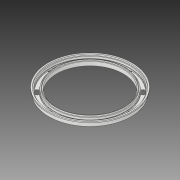
# Autodesk Inventor part: led_holster
Saved by Autodesk Inventor 2019.3 (Build 233278000, 278)
## iProperties
Created: 2019-03-01
Part Number: led_holster
Material: ABS Plastic
Document SubType Name: Modeling
Designer: WW
Density: 1.06 g/cm^3
Appearance: Smooth - White
Author: WW
Autodesk Inventor part; units mm, degrees
ref_plane "YZ Plane" through (0, 0, 0) normal (1, 0, 0) x (0, 1, 0)
ref_plane "XZ Plane" through (0, 0, 0) normal (0, 1, 0) x (-1, 0, 0)
ref_plane "XY Plane" through (0, 0, 0) normal (0, 0, 1) x (1, 0, 0)
sketch "Sketch1" plane through (0, 0, 0) normal (0, 0, 1) x (1, 0, 0)
  line L0 (0, 0) -> (0, -5) construction
  line L1 (78, 0) -> (78, -3.2)
  line L2 (92, -3.2) -> (92, 0)
  line L3 (90, -3.2) -> (90, -7.7)
  line L4 (90, -7.7) -> (80, -7.7) construction
  line L5 (80, -7.7) -> (80, -3.2)
  line L6 (78, -3.2) -> (80, -3.2)
  line L7 (90, -3.2) -> (92, -3.2)
  line L8 (81, -7.7) -> (89, -7.7) construction
  line L9 (89, -7.7) -> (89, -10.1)
  line L10 (89, -10.1) -> (81, -10.1) construction
  line L11 (81, -10.1) -> (81, -7.7)
  line L12 (81, -10.1) -> (77, -10.1)
  line L13 (77, -10.1) -> (77, 0)
  line L14 (77, 0) -> (78, 0)
  line L15 (78, 0) -> (92, 0) construction
  line L16 (85, 0) -> (85, 0.6686) construction
  line L17 (89, -10.1) -> (93, -10.1)
  line L18 (93, -10.1) -> (93, 0)
  line L19 (93, 0) -> (92, 0)
  line L20 (80, -7.7) -> (81, -7.7)
  line L21 (89, -7.7) -> (90, -7.7)
  line L22 (77, -10.1) -> (93, -10.1)
  line L23 (93, -10.1) -> (93, -11.3)
  line L24 (93, -11.3) -> (77, -11.3)
  line L25 (77, -11.3) -> (77, -10.1)
  point P0 (85, -7.7)
  dimension "d0" = 5
  dimension "d1" = 3.2
  dimension "d4" = 1
  dimension "d5" = 10
  dimension "d6" = 4.5
  dimension "d7" = 2.4
  dimension "d8" = 1
  dimension "d9" = 170
  dimension "d10" = 2
  dimension "d12" = 1.2
  constraints: 52 end point, 10 perpendicular, 7 horizontal, 5 parallel, 4 vertical, 3 collinear, 3 horizontal alignment, 3 midpoint, 1 point on line
  measures "d0" distance of L0.start L0.end
  measures "d1" distance from line of L1.start L6
  measures "d4" distance between parallel lines of L1 L13
  measures "d5" distance of L3.end L4.end
  measures "d6" distance of L3.start L3.end
  measures "d7" distance between parallel lines of L12 L4
  measures "d8" distance from line of L9 L3.end
  measures "d9" diameter of L16 L0
  measures "d10" distance of L1.end L5.end
  measures "d12" distance of L24.end L12.end
revolve "Revolution1" add sketch "Sketch1" angle 360 about axis through (0, 0, 0) along (0, -1, 0)
sketch "Sketch2" plane through (0, -10.1, 0) normal (0, 1, 0) x (1, 0, 0)
  circle A0 centre (0, 0) radius 89 construction
  circle A1 centre (0, 0) radius 81 construction
  arc A2 (-7.6914, -88.667) -> (7.6914, -88.667) centre (0, 0) ccw
  arc A3 (-7, -80.697) -> (7, -80.697) centre (0, 0) ccw
  line L0 (-7.6914, -88.667) -> (-7, -80.697)
  line L1 (7, -80.697) -> (7.6914, -88.667)
  line L2 (-7, -80.697) -> (7, -80.697) construction
  point P0 (0, -80.697)
  dimension "d14" = 14
  constraints: 8 point on circle, 6 end point, 2 centre point, 2 concentric, 2 line through centre, 1 midpoint, 1 vertical alignment
  measures "d14" distance of L1.start L0.end
extrude "Extrusion1" cut sketch "Sketch2" against normal through all
fillet "Fillet1" radius 3 4 edges at (-7.6914, -10.7, 88.667) (7.6914, -10.7, 88.667) (-7, -10.7, 80.697) (7, -10.7, 80.697)
pattern_circular "Circular Pattern1" count 8 over 360 about axis through (0, -5.05, 0) along (0, -1, 0) of "Extrusion1", "Fillet1"
sketch "Sketch4" plane through (0, -11.3, 0) normal (0, -1, 0) x (1, 0, 0)
  circle A0 centre (0, 0) radius 77 projected
  circle A1 centre (0, 0) radius 75
  dimension "d27" = 2
  constraints: 1 centre point
  measures "d27" radial gap between concentric circles of A0 A1
extrude "Extrusion3" add sketch "Sketch4" against normal blind 8.8
sketch "Sketch5" plane through (0, 0, 0) normal (0, 1, 0) x (1, 0, 0)
  circle A0 centre (0, 0) radius 93 projected
  circle A1 centre (0, 0) radius 95
  dimension "d30" = 2
  constraints: 1 centre point
  measures "d30" radial gap between concentric circles of A0 A1
extrude "Extrusion4" add sketch "Sketch5" against normal blind 2.5
body "Solid1"
